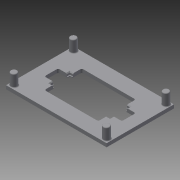
# Autodesk Inventor part: 1x3 slide SD stage insert large clearance
Saved by Autodesk Inventor 2013 (Build 170138000, 138)
## iProperties
Created: 2012-10-15
Part Number: 1x3 slide SD stage insert large clearance
Material: Generic
Document SubType Name: Modeling
Designer: kthorn
Density: 1 g/cm^3
Author: kthorn
Autodesk Inventor part; units mm, degrees
ref_plane "YZ Plane" through (0, 0, 0) normal (1, 0, 0) x (0, 1, 0)
ref_plane "XZ Plane" through (0, 0, 0) normal (0, 1, 0) x (-1, 0, 0)
ref_plane "XY Plane" through (0, 0, 0) normal (0, 0, 1) x (1, 0, 0)
sketch "Sketch1" plane through (0, 0, 0) normal (0, 0, 1) x (1, 0, 0)
  line L0 (-63.85, 42.75) -> (63.85, 42.75)
  line L1 (63.85, 42.75) -> (63.85, -42.75)
  line L2 (63.85, -42.75) -> (-63.85, -42.75)
  line L3 (-63.85, -42.75) -> (-63.85, 42.75)
  line L4 (-63.85, 42.75) -> (63.85, -42.75) construction
  line L5 (63.85, 42.75) -> (-63.85, -42.75) construction
  point P0 (0, 0)
  dimension "d0" = 127.7
  dimension "d1" = 85.5
  constraints: 12 end point, 2 midpoint, 2 parallel, 1 horizontal, 1 perpendicular
  measures "d0" distance of L1.end L2.end
  measures "d1" distance of L0.end L1.end
extrude "Extrusion1" add sketch "Sketch1" along normal blind 4.5
sketch "Sketch2" plane through (0, 0, 4.5) normal (0, 0, 1) x (1, 0, 0)
  line L0 (-38.25, 12.75) -> (38.25, 12.75)
  line L1 (38.25, 12.75) -> (38.25, -12.75)
  line L2 (38.25, -12.75) -> (-38.25, -12.75)
  line L3 (-38.25, -12.75) -> (-38.25, 12.75)
  line L4 (-38.25, 12.75) -> (38.25, -12.75) construction
  line L5 (38.25, 12.75) -> (-38.25, -12.75) construction
  point P0 (0, 0)
  dimension "d4" = 76.5
  dimension "d5" = 25.5
  constraints: 12 end point, 2 midpoint, 2 parallel, 1 horizontal, 1 perpendicular
  measures "d4" distance of L1.end L2.end
  measures "d5" distance of L0.end L1.end
extrude "Extrusion2" cut sketch "Sketch2" against normal blind 3.5
sketch "Sketch3" plane through (0, 0, 1) normal (0, 0, 1) x (1, 0, 0)
  line L0 (-38.25, 12.75) -> (38.25, 12.75) projected
  line L1 (38.25, 12.75) -> (38.25, -12.75) projected
  line L2 (-37.25, 11.75) -> (37.25, 11.75)
  line L3 (37.25, 11.75) -> (37.25, -11.75)
  line L4 (37.25, -11.75) -> (-37.25, -11.75)
  line L5 (-37.25, -11.75) -> (-37.25, 11.75)
  line L6 (-37.25, 11.75) -> (37.25, -11.75) construction
  line L7 (37.25, 11.75) -> (-37.25, -11.75) construction
  line L8 (0, 11.75) -> (0, 12.75) construction
  line L9 (37.25, 0) -> (38.25, 0) construction
  point P0 (0, 0)
  dimension "d8" = 1
  constraints: 16 end point, 6 midpoint, 2 parallel, 2 perpendicular, 1 horizontal
  measures "d8" distance of L8.start L8.end
extrude "Extrusion3" cut sketch "Sketch3" against normal through all
chamfer "Chamfer1" distance 1 angle 45 4 edges at (-38.25, 0, 4.5) (0, 12.75, 4.5) (38.25, 0, 4.5) (0, -12.75, 4.5)
sketch "Sketch4" plane through (0, 0, 4.5) normal (0, 0, 1) x (1, 0, 0)
  line L0 (63.85, 42.75) -> (-63.85, 42.75) projected
  circle A0 centre (-58.85, 37.75) radius 4
  line L1 (-63.85, 42.75) -> (-58.85, 42.75) construction
  line L2 (-58.85, 42.75) -> (-58.85, 37.75) construction
  line L3 (-63.85, 42.75) -> (-63.85, -42.75) projected
  line L4 (-63.85, -42.75) -> (63.85, -42.75) projected
  line L5 (63.85, -42.75) -> (63.85, 42.75) projected
  line L6 (0, 42.75) -> (0, -42.75) construction
  line L7 (-63.85, 0) -> (63.85, 0) construction
  circle A1 centre (58.85, 37.75) radius 4
  circle A2 centre (-58.85, -37.75) radius 4
  circle A3 centre (58.85, -37.75) radius 4
  point P0 (0, 0)
  dimension "d15" = 8
  dimension "d17" = 5
  constraints: 8 end point, 4 centre point, 4 midpoint, 3 symmetric about line, 2 perpendicular, 1 coincident, 1 point on line, 3 other
  measures "d15" diameter of A0
  measures "d17" distance of L1.end L2.end
extrude "Extrusion4" add sketch "Sketch4" along normal blind 15 contours A0 | A1 | A2 | A3
fillet "Fillet1" radius 1 8 edges at (-62.85, 37.75, 19.5) (-62.85, 37.75, 4.5) (-62.85, -37.75, 19.5) (-62.85, -37.75, 4.5) (54.85, 37.75, 19.5) (54.85, 37.75, 4.5) (54.85, -37.75, 19.5) (54.85, -37.75, 4.5)
sketch "Sketch5" plane through (0, 0, 4.5) normal (0, 0, 1) x (1, 0, 0)
  line L0 (-39.25, 13.75) -> (-39.25, -13.75) projected
  line L1 (39.25, 13.75) -> (-39.25, 13.75) projected
  line L2 (34.25, -23.75) -> (-34.25, -23.75)
  line L3 (-34.25, -23.75) -> (-34.25, 23.75)
  line L4 (-34.25, 23.75) -> (34.25, 23.75)
  line L5 (34.25, 23.75) -> (34.25, -23.75)
  line L6 (34.25, -23.75) -> (-34.25, 23.75) construction
  line L7 (-34.25, -23.75) -> (34.25, 23.75) construction
  line L8 (-49.25, -8.75) -> (49.25, -8.75)
  line L9 (49.25, -8.75) -> (49.25, 8.75)
  line L10 (49.25, 8.75) -> (-49.25, 8.75)
  line L11 (-49.25, 8.75) -> (-49.25, -8.75)
  line L12 (-49.25, -8.75) -> (49.25, 8.75) construction
  line L13 (49.25, -8.75) -> (-49.25, 8.75) construction
  line L14 (34.25, 23.75) -> (34.25, 13.75) construction
  line L15 (-34.25, 13.75) -> (-39.25, 13.75) construction
  line L16 (-39.25, -8.75) -> (-39.25, -13.75) construction
  line L17 (-39.25, 8.75) -> (-49.25, 8.75) construction
  line L18 (-39.25, 8.75) -> (-49.25, 8.75) construction
  point P0 (0, 0)
  dimension "d22" = 10
  dimension "d24" = 5
  dimension "d25" = 5
  dimension "d26" = 10
  constraints: 34 end point, 8 point on line, 4 collinear, 4 midpoint, 4 parallel, 2 horizontal, 2 perpendicular
  measures "d22" distance of L4.end L14.end
  measures "d24" distance of L15.start L0.start
  measures "d25" distance of L16.start L0.end
  measures "d26" distance of L17.start L10.end
extrude "Extrusion5" cut sketch "Sketch5" against normal through all contours L10 L3 L8 L0 | L0 L8 L11 L10 | L3 L4 L5 L1 | L1 L5 L10 L3 | L10 L5 L8 L3 | L8 L5 L2 L3 | L10 L9 L8 L5
fillet "Fillet2" radius 2 8 edges at (34.25, -23.75, 2.25) (49.25, -8.75, 2.25) (49.25, 8.75, 2.25) (34.25, 23.75, 2.25) (-34.25, 23.75, 2.25) (-49.25, 8.75, 2.25) (-34.25, -23.75, 2.25) (-49.25, -8.75, 2.25)
body "Solid1"
